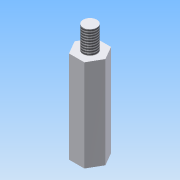
# Autodesk Inventor part: 서포터 20
Saved by Autodesk Inventor 2015 (Build 190159000, 159)
## iProperties
Created: 2013-09-16
Part Number: 서포터 20
Material: 일반
Document SubType Name: Modeling
Designer: Jeong
Density: 1 g/cm^3
Mass: 0.582662 g
Surface Area: 5.5435 cm^2
Volume: 0.582662 cm^3
Appearance: PTFE
Author: Jeong
Autodesk Inventor part; units mm, degrees
ref_plane "YZ Plane" through (0, 0, 0) normal (1, 0, 0) x (0, 1, 0)
ref_plane "XZ Plane" through (0, 0, 0) normal (0, 1, 0) x (-1, 0, 0)
ref_plane "XY Plane" through (0, 0, 0) normal (0, 0, 1) x (1, 0, 0)
sketch "스케치1" plane through (0, 0, 0) normal (0, 0, 1) x (1, 0, 0)
  line L0 (1.6743, 2.9) -> (3.3486, 0)
  line L1 (3.3486, 0) -> (1.6743, -2.9)
  line L2 (1.6743, -2.9) -> (-1.6743, -2.9)
  line L3 (-1.6743, -2.9) -> (-3.3486, 0)
  line L4 (-3.3486, 0) -> (-1.6743, 2.9)
  line L5 (-1.6743, 2.9) -> (1.6743, 2.9)
  point P0 (0, 0)
  constraints: 12 end point, 13 other
extrude "돌출1" add sketch "스케치1" along normal blind 20
sketch "스케치2" plane through (0, 0, 20) normal (0, 0, 1) x (1, 0, 0)
  circle A0 centre (0, 0) radius 1.5
  dimension "d6" = 3
  constraints: 1 centre point, 1 coincident
  measures "d6" diameter of A0
extrude "돌출2" add sketch "스케치2" along normal blind 5
thread "스레드1" size "M3x0.5" class "6g" standard "ANSI Metric M Profile" full length
sketch "스케치3" plane through (0, 0, 0) normal (0, 0, -1) x (-1, 0, 0)
  circle A0 centre (0, 0) radius 1.5
  dimension "d11" = 3
  constraints: 1 centre point, 1 coincident
  measures "d11" diameter of A0
extrude "돌출3" cut sketch "스케치3" against normal blind 5
thread "스레드2" size "M3x0.5" class "6H" standard "ANSI Metric M Profile" full length
